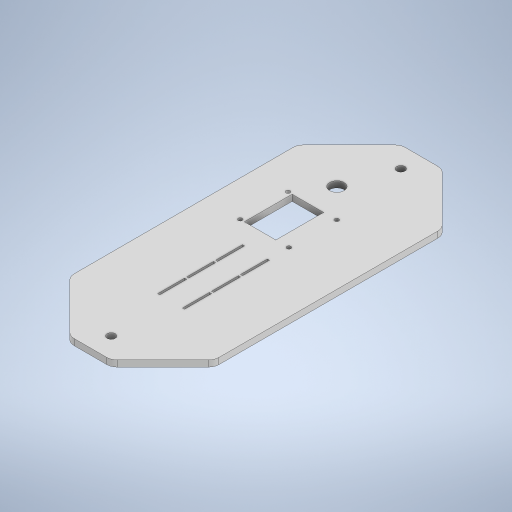
# Autodesk Inventor part: panel
Saved by Autodesk Inventor 2024.4 (Build 284460000, 460)
## iProperties
Created: 2026-03-15
Part Number: panel
Material: Generic
Document SubType Name: Modeling
Designer: HP
Density: 1 g/cm^3
Appearance: Default
Author: HP
Autodesk Inventor part; units mm, degrees
ref_plane "YZ Plane" through (0, 0, 0) normal (1, 0, 0) x (0, 1, 0)
ref_plane "XZ Plane" through (0, 0, 0) normal (0, 1, 0) x (-1, 0, 0)
ref_plane "XY Plane" through (0, 0, 0) normal (0, 0, 1) x (1, 0, 0)
sketch "Sketch1" plane through (0, 0, 0) normal (0, 1, 0) x (-1, 0, 0)
  line L0 (0, 0) -> (0, 80)
  line L1 (0, 80) -> (0, -80)
  line L2 (0, 80) -> (35, 80)
  line L3 (35, 80) -> (35, -80)
  line L4 (35, -80) -> (-35, -80)
  line L5 (-35, -80) -> (-35, 80)
  line L6 (-35, 80) -> (0, 80)
  line L7 (0, 80) -> (10, 80)
  line L8 (35, 80) -> (35, 55)
  line L9 (10, 80) -> (35, 55)
  line L10 (35, 0) -> (-35, 0)
  line L11 (0, 80) -> (0, -80)
  line L12 (10, -80) -> (35, -55)
  line L13 (-10, 80) -> (-35, 55)
  line L14 (-10, -80) -> (-35, -55)
  line L15 (0, 0) -> (0, 70)
  line L16 (0, 70) -> (0, -70)
  circle A0 centre (0, 70) radius 2
  circle A1 centre (0, -70) radius 2
  dimension "d0" = 80
  dimension "d1" = 160
  dimension "d2" = 35
  dimension "d3" = 70
  dimension "d4" = 10
  dimension "d5" = 25
  dimension "d6" = 70
  dimension "d7" = 140
  dimension "d8" = 4
  dimension "d9" = 4
  constraints: 34 end point, 6 point on line, 6 symmetric about line, 5 perpendicular, 2 centre point, 2 coincident, 2 midpoint, 1 horizontal, 1 vertical
  measures "d0" distance of L0.start L0.end
  measures "d1" distance of L0.end L1.end
  measures "d2" distance of L0.end L2.end
  measures "d3" distance of L3.end L4.end
  measures "d4" distance of L0.end L7.end
  measures "d5" distance of L2.end L8.end
  measures "d6" distance of L0.start L15.end
  measures "d7" distance of L15.end L16.end
  measures "d8" diameter of A0
  measures "d9" diameter of A1
extrude "Extrusion1" add sketch "Sketch1" along normal blind 3 contours L10 L5 L13 L6 L0 A0 | L10 L3 L12 L4 L1 A1 | L0 A0 L2 L9 L3 L10 | L1 A1 L4 L14 L5 L10
fillet "Fillet1" radius 5 8 edges at (-35, 1.5, 55) (-10, 1.5, 80) (-35, 1.5, -55) (35, 1.5, 55) (10, 1.5, 80) (35, 1.5, -55) (10, 1.5, -80) (-10, 1.5, -80)
sketch "Sketch2" plane through (0, 3, 0) normal (0, 1, 0) x (1, 0, 0)
  line L0 (0, 0) -> (0, 10)
  line L1 (5.9101, 10) -> (-17.6499, 10)
  line L2 (-17.6499, 10) -> (-17.6499, 33.1)
  line L3 (-17.6499, 33.1) -> (5.9101, 33.1)
  line L4 (5.9101, 33.1) -> (5.9101, 10)
  line L5 (0, 10) -> (0, 21.55)
  line L6 (0, 21.55) -> (20, 21.55)
  line L7 (35, -52.9289) -> (35, 52.9289) projected
  circle A0 centre (20, 21.55) radius 3.5
  circle A1 centre (-17.6499, 10) radius 1
  circle A2 centre (-17.6499, 33.1) radius 1
  circle A3 centre (5.9101, 10) radius 1
  circle A4 centre (5.9101, 33.1) radius 1
  line L8 (0, 0) -> (-6, 0)
  line L9 (-6, 0) -> (-6, -50)
  line L10 (-6, -50) -> (6, -50)
  line L11 (6, -50) -> (6, 0)
  line L12 (6, 0) -> (-6, 0)
  line L13 (-6, -50) -> (-6.5, -50)
  line L14 (-6.5, -50) -> (-6.5, 0)
  line L15 (-6.5, 0) -> (-5.5, 0)
  line L16 (-5.5, 0) -> (-5.5, -50)
  line L17 (-5.5, -50) -> (-6.5, -50)
  line L18 (0, 0) -> (0, -66.8235)
  line L19 (6, -50) -> (6.5, -50)
  line L20 (6.5, -50) -> (6.5, 0)
  line L21 (6.5, 0) -> (5.5, 0)
  line L22 (5.5, 0) -> (5.5, -50)
  line L23 (5.5, -50) -> (6.5, -50)
  line L24 (0, 21.55) -> (6, 21.55)
  dimension "d13" = 10
  dimension "d14" = 23.56
  dimension "d15" = 23.1
  dimension "d16" = 11.55
  dimension "d17" = 20
  dimension "d18" = 7
  dimension "d19" = 2
  dimension "d20" = 2
  dimension "d21" = 2
  dimension "d22" = 2
  dimension "d23" = 6
  dimension "d24" = 50
  dimension "d25" = 12
  dimension "d26" = 0.5
  dimension "d27" = 1
  dimension "d37" = 6
  constraints: 48 end point, 8 perpendicular, 5 centre point, 5 coincident, 5 point on line, 4 symmetric about line, 3 vertical, 2 collinear, 2 horizontal
  measures "d13" distance of L0.end L0.start
  measures "d14" distance of L1.start L1.end
  measures "d15" distance of L1.end L2.end
  measures "d16" distance of L5.start L5.end
  measures "d17" distance of L5.end L6.end
  measures "d18" diameter of A0
  measures "d19" diameter of A1
  measures "d20" diameter of A2
  measures "d21" diameter of A3
  measures "d22" diameter of A4
  measures "d23" distance of L0.start L8.end
  measures "d24" distance of L8.end L9.end
  measures "d25" distance of L9.end L10.end
  measures "d26" distance of L9.end L13.end
  measures "d27" distance of L14.end L15.end
  measures "d37" distance of L5.end L24.end
extrude "Extrusion2" cut sketch "Sketch2" against normal blind 10 contours A0 | L16 L10 L9 L8 | L12 L11 L10 L22 | A1 L2 L1 | L1 L2 A1 | A3 L4 L1 | L1 L4 A3 | L9 L13 L14 L15 | L21 L20 L19 L11 | A2 L3 L2 | L2 L3 A2 | A4 L3 L4 | L4 L3 A4
sketch "Sketch3" plane through (0, 3, 0) normal (0, 1, 0) x (1, 0, 0)
  line L0 (-5.5, -50) -> (-5.5, 0) projected
  line L1 (-5.5, 0) -> (-5.5, -13)
  line L2 (-5.5, -13) -> (-6.5, -13)
  line L3 (-6.5, -50) -> (-6.5, 0) projected
  line L4 (-6.5, 0) -> (-6.5, -13)
  line L5 (-6.5, 0) -> (-5.5, 0)
  line L6 (-6.5, -13) -> (-6.5, -14)
  line L7 (-6.5, -14) -> (-5.5, -14)
  line L8 (-5.5, -14) -> (-5.5, -13)
  line L9 (-6.5, -13) -> (-5.5, -13)
  line L10 (-6.5, -14) -> (-6.5, -27)
  line L11 (-6.5, -27) -> (-6.5, -28)
  line L12 (-6.5, -28) -> (-5.5, -28)
  line L13 (-5.5, -28) -> (-5.5, -27)
  line L14 (-5.5, -27) -> (-6.5, -27)
  line L15 (-5.5, -14) -> (-5.5, -27)
  line L16 (-6.5, -28) -> (-6.5, -41)
  line L17 (-6.5, -41) -> (-5.5, -41)
  line L18 (-5.5, -41) -> (-5.5, -28)
  line L19 (-6.5, -28) -> (-5.5, -28)
  line L20 (-6.5, -50) -> (-5.5, -50) projected
  line L21 (-6.5, -41) -> (-6.5, -50)
  line L22 (-6.5, -50) -> (-5.5, -50)
  line L23 (-5.5, -50) -> (-5.5, -41)
  line L24 (0, 0) -> (0, -62.7524)
  line L25 (5.5, -50) -> (5.5, 0)
  line L26 (5.5, -13) -> (6.5, -13)
  line L27 (6.5, -50) -> (6.5, 0)
  line L28 (6.5, 0) -> (5.5, 0)
  line L29 (6.5, -14) -> (5.5, -14)
  line L30 (6.5, -28) -> (5.5, -28)
  line L31 (5.5, -27) -> (6.5, -27)
  line L32 (6.5, -41) -> (5.5, -41)
  line L33 (6.5, -50) -> (5.5, -50)
  dimension "d30" = 13
  dimension "d31" = 1
  dimension "d32" = 13
  dimension "d33" = 1
  dimension "d34" = 13
  constraints: 62 end point, 14 symmetric about line, 13 point on line, 9 perpendicular, 6 collinear, 1 vertical
  measures "d30" distance of L0.end L1.end
  measures "d31" distance of L2.end L6.end
  measures "d32" distance of L6.end L10.end
  measures "d33" distance of L10.end L11.end
  measures "d34" distance of L11.end L16.end
extrude "Extrusion3" add sketch "Sketch3" against normal blind 3 contours L20 L3 L17 L0 | L12 L3 L14 L0 | L7 L3 L2 L0 | L25 L32 L27 L33 | L25 L31 L27 L30 | L25 L26 L27 L29
sketch "Sketch4" plane through (0, 3, 0) normal (0, 1, 0) x (1, 0, 0)
  circle A0 centre (-17.6499, 10) radius 1 projected
  line L0 (-17.6499, 10) -> (-15.6499, 10)
  circle A1 centre (-17.6499, 33.1) radius 1 projected
  line L1 (-17.6499, 33.1) -> (-15.6499, 33.1)
  line L2 (-15.6499, 10) -> (-15.6499, 33.1)
  circle A2 centre (5.9101, 33.1) radius 1 projected
  line L3 (5.9101, 33.1) -> (-0.3899, 33.1)
  circle A3 centre (5.9101, 10) radius 1 projected
  line L4 (5.9101, 10) -> (-0.3899, 10)
  line L5 (-15.6499, 10) -> (-0.3899, 10)
  line L6 (-0.3899, 10) -> (-0.3899, 33.1)
  line L7 (-0.3899, 33.1) -> (-15.6499, 33.1)
  point P0 (0, 0)
  dimension "d38" = 2
  dimension "d39" = 2
  dimension "d40" = 6.3
  dimension "d41" = 6.3
  constraints: 16 end point, 4 horizontal, 1 collinear
  measures "d38" distance of L0.start L0.end
  measures "d39" distance of L1.start L1.end
  measures "d40" distance of L3.start L3.end
  measures "d41" distance of L4.start L4.end
extrude "Extrusion4" cut sketch "Sketch4" against normal blind 10 contours L2 L7 L6 L5
sketch "Sketch5" plane through (0, 3, 0) normal (0, 1, 0) x (1, 0, 0)
  circle A0 centre (20, 21.55) radius 3.5 projected
  circle A1 centre (20, 21.55) radius 3.5
  point P0 (0, 0)
  constraints: 1 centre point, 1 coincident
extrude "Extrusion5" add sketch "Sketch5" against normal blind 3
sketch "Sketch6" plane through (0, 3, 0) normal (0, 1, 0) x (1, 0, 0)
  line L0 (0, 0) -> (0, 62.477)
  line L1 (-15.6499, 33.1) -> (-0.3899, 33.1) projected
  line L2 (-8.0199, 33.1) -> (-8.0199, 54.1)
  line L3 (-8.0199, 54.1) -> (0, 54.1)
  line L4 (-8.0199, 33.1) -> (-8.0199, 41.1)
  line L5 (-8.0199, 33.1) -> (-8.0199, 47.1)
  circle A0 centre (-8.0199, 47.1) radius 3.5
  dimension "d46" = 21
  dimension "d47" = 8
  dimension "d48" = 14
  dimension "d49" = 7
  constraints: 10 end point, 3 point on line, 2 vertical, 1 centre point, 1 coincident, 1 midpoint, 1 perpendicular
  measures "d46" distance of L2.start L2.end
  measures "d47" distance of L2.start L4.end
  measures "d48" distance of L2.start L5.end
  measures "d49" diameter of A0
extrude "Extrusion6" cut sketch "Sketch6" against normal blind 3
body "Solid1"
